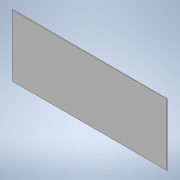
# Autodesk Inventor part: ChassisWall
Saved by Autodesk Inventor 2020 (Build 240168000, 168)
## iProperties
Created: 2021-11-11
Part Number: ChassisWall
Material: Generic
Document SubType Name: Modeling
Designer: 17185
Density: 1 g/cm^3
Appearance: Default
Author: 17185
Autodesk Inventor part; units mm, degrees
ref_plane "YZ Plane" through (0, 0, 0) normal (1, 0, 0) x (0, 1, 0)
ref_plane "XZ Plane" through (0, 0, 0) normal (0, 1, 0) x (-1, 0, 0)
ref_plane "XY Plane" through (0, 0, 0) normal (0, 0, 1) x (1, 0, 0)
sketch "Sketch1" plane through (0, 0, 0) normal (0, 0, 1) x (1, 0, 0)
  line L0 (-381, 152.4) -> (381, 152.4)
  line L1 (381, 152.4) -> (381, -152.4)
  line L2 (381, -152.4) -> (-381, -152.4)
  line L3 (-381, -152.4) -> (-381, 152.4)
  line L4 (-381, 152.4) -> (381, -152.4) construction
  line L5 (381, 152.4) -> (-381, -152.4) construction
  point P0 (0, 0)
  dimension "d0" = 762
  dimension "d1" = 304.8
  constraints: 12 end point, 2 midpoint, 2 parallel, 1 horizontal, 1 perpendicular
  measures "d0" distance of L0.start L0.end
  measures "d1" distance of L0.end L1.end
extrude "Extrusion1" add sketch "Sketch1" along normal blind 3.175
body "Solid1"
